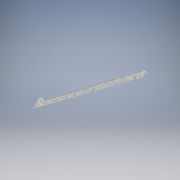
# Autodesk Inventor part: アーム先端1
Saved by Autodesk Inventor 2020 (Build 240168000, 168)
## iProperties
Created: 2018-11-26
Part Number: アーム先端1
Material: アルミニウム 7075
Document SubType Name: Modeling
Designer: 雪村
Density: 2.81 g/cm^3
Appearance: サテン - ブラシ仕上げ 重厚
Mass: 28.3471 g
Surface Area: 102.55 cm^2
Volume: 10.0879 cm^3
Description: アルミ7000 6t
Author: 雪村
Autodesk Inventor part; units mm, degrees
ref_plane "YZ Plane" through (0, 0, 0) normal (1, 0, 0) x (0, 1, 0)
ref_plane "XZ Plane" through (0, 0, 0) normal (0, 1, 0) x (-1, 0, 0)
ref_plane "XY Plane" through (0, 0, 0) normal (0, 0, 1) x (1, 0, 0)
sketch "スケッチ1" plane through (0, 0, 0) normal (0, 0, 1) x (1, 0, 0)
  line L0 (-218.2218, -75.2242) -> (-181.0358, -47.3081)
  line L1 (-181.0358, -47.3081) -> (-413.1791, -221.5813)
  line L2 (-39.9318, 79.9092) -> (-423.8001, -208.2662) construction
  arc A0 (-413.8727, -220.8729) -> (-413.1791, -221.5813) centre (-413.4792, -221.1815) ccw
  line L3 (-413.8727, -220.8729) -> (-401.6494, -205.2862)
  line L4 (-401.6494, -205.2862) -> (-186.2425, -41.2134)
  line L5 (-181.4863, -40.7689) -> (-171.6699, -53.845) construction
  line L6 (-423.8001, -208.2662) -> (-390.8364, -252.1761) construction
  circle A1 centre (-209.3341, -63.7077) radius 1.5
  circle A2 centre (-183.8101, -44.4068) radius 1.5
  arc A3 (-181.0358, -47.3081) -> (-186.2425, -41.2134) centre (-183.8101, -44.4068) ccw
  point P0 (0, 0)
  point P1 (0, 0)
  dimension "d0" = 1
  dimension "d1" = 15
  dimension "d2" = 8
  dimension "d3" = 0.4
  constraints: 14 end point, 4 centre point, 4 point on circle, 4 tangent, 1 parallel, 1 perpendicular, 6 other
  measures "d0" diameter of A0
  measures "d1" angle of L1 L3
  measures "d2" distance from line of L0 L4.end
  measures "d3" angle of L1 L4
extrude "押し出し1" add sketch "スケッチ1" along normal blind 6
sketch "スケッチ2" plane through (0, 0, 6) normal (0, 0, 1) x (1, 0, 0)
  circle A0 centre (-183.8101, -44.4068) radius 1.5 projected
  circle A1 centre (-209.3341, -63.7077) radius 1.5 projected
  line L0 (-413.1791, -221.5813) -> (-181.0358, -47.3081) projected
  arc A2 (-181.0358, -47.3081) -> (-186.2425, -41.2134) centre (-183.8101, -44.4068) ccw projected
  line L1 (-186.2425, -41.2134) -> (-401.6494, -205.2862) projected
  line L2 (-401.6494, -205.2862) -> (-413.8727, -220.8729) projected
  arc A3 (-413.8727, -220.8729) -> (-413.1791, -221.5813) centre (-413.4792, -221.1815) ccw projected
  line L3 (-183.8101, -44.4068) -> (-185.0065, -45.3115)
  line L4 (-209.7841, -65.1386) -> (-419.2967, -222.4226) construction
  line L5 (-413.1791, -221.5813) -> (-181.0358, -47.3081) projected
  circle A4 centre (-399.7939, -207.7816) radius 1.5
  circle A5 centre (-379.8007, -192.7724) radius 1.5
  circle A6 centre (-359.8076, -177.7633) radius 1.5
  circle A7 centre (-339.8144, -162.7542) radius 1.5
  circle A8 centre (-319.8213, -147.745) radius 1.5
  circle A9 centre (-299.8281, -132.7359) radius 1.5
  circle A10 centre (-399.7939, -207.7816) radius 3 construction
  line L6 (-401.6494, -205.2862) -> (-413.8727, -220.8729) projected
  circle A11 centre (-283.8336, -120.7286) radius 1.5
  circle A12 centre (-263.8405, -105.7194) radius 1.5
  circle A13 centre (-223.8542, -75.7012) radius 1.5
  circle A14 centre (-243.8473, -90.7103) radius 1.5
  point P0 (0, 0)
  dimension "d6" = 3
  dimension "d7" = 3
  dimension "d8" = 3
  dimension "d9" = 3
  dimension "d10" = 3
  dimension "d11" = 3
  dimension "d12" = 3
  dimension "d15" = 25
  dimension "d16" = 25
  dimension "d17" = 25
  dimension "d18" = 25
  dimension "d19" = 25
  dimension "d50" = 3
  dimension "d51" = 3
  dimension "d52" = 3
  dimension "d53" = 3
  dimension "d55" = 25
  dimension "d56" = 25
  dimension "d57" = 25
  dimension "d61" = 20
  constraints: 11 centre point, 2 end point, 2 tangent, 18 other
  measures "d7" diameter of A4
  measures "d8" diameter of A5
  measures "d9" diameter of A6
  measures "d10" diameter of A7
  measures "d11" diameter of A8
  measures "d12" diameter of A9
  measures "d15" distance of A5.centre A4.centre
  measures "d16" distance of A6.centre A5.centre
  measures "d17" distance of A7.centre A6.centre
  measures "d18" distance of A8.centre A7.centre
  measures "d19" distance of A8.centre A9.centre
  measures "d50" diameter of A11
  measures "d51" diameter of A12
  measures "d52" diameter of A13
  measures "d53" diameter of A14
  measures "d55" distance of A12.centre A11.centre
  measures "d56" distance of A14.centre A12.centre
  measures "d57" distance of A14.centre A13.centre
  measures "d61" distance of A9.centre A11.centre
extrude "押し出し2" cut sketch "スケッチ2" against normal blind 10 contours A4 | A5 | A6 | A7 | A8 | A9 | A11 | A12 | A13 | A14
sketch "スケッチ7" plane through (0, 0, 6) normal (0, 0, 1) x (1, 0, 0)
  line L0 (-413.1791, -221.5813) -> (-181.0358, -47.3081) construction
  arc A0 (-181.0358, -47.3081) -> (-186.2425, -41.2134) centre (-183.8101, -44.4068) ccw construction
  line L1 (-186.2425, -41.2134) -> (-401.6494, -205.2862) construction
  line L2 (-401.6494, -205.2862) -> (-413.8727, -220.8729) projected
  arc A1 (-413.8727, -220.8729) -> (-413.1791, -221.5813) centre (-413.4792, -221.1815) ccw projected
  circle A2 centre (-209.3341, -63.7077) radius 1.5 construction
  circle A3 centre (-183.8101, -44.4068) radius 1.5 construction
  line L3 (-186.2425, -41.2134) -> (-401.6494, -205.2862) projected
  line L4 (-401.6494, -205.2862) -> (-413.8727, -220.8729) projected
  line L5 (-413.9292, -220.9634) -> (-400.843, -193.968)
  arc A4 (-400.843, -193.968) -> (-394.0669, -199.5107) centre (-396.7936, -195.9309) ccw
  arc A5 (-413.8727, -220.8729) -> (-413.1791, -221.5813) centre (-413.4792, -221.1815) ccw projected
  point P0 (0, 0)
  dimension "d45" = 9
  dimension "d46" = 30
  constraints: 3 point on circle, 3 tangent, 2 end point, 1 centre point, 1 point on line
  measures "d45" diameter of A4
  measures "d46" distance of L5.start L5.end
extrude "押し出し6" add sketch "スケッチ7" against normal blind 6
fillet "フィレット3" radius 1 1 edges at (-400.843, -193.968, 3)
sketch "スケッチ13" plane through (0, 0, 6) normal (0, 0, 1) x (1, 0, 0)
  circle A0 centre (-183.8101, -44.4068) radius 1.5 construction
  circle A1 centre (-399.7939, -207.7816) radius 1.5 projected
  circle A2 centre (-183.8101, -44.4068) radius 1.5 construction
  line L0 (-185.6423, -44.4646) -> (-186.6877, -45.2549) construction
  circle A3 centre (-399.7939, -207.7816) radius 1.5 projected
  line L1 (-397.9939, -207.6808) -> (-396.933, -206.8784) construction
  line L2 (-185.6423, -44.4646) -> (-184.3878, -46.1357) construction
  line L3 (-413.1791, -221.5813) -> (-181.0358, -47.3081) construction
  line L4 (-399.2667, -205.9854) -> (-397.9939, -207.6808) construction
  line L5 (-186.2425, -41.2134) -> (-394.0669, -199.5107) construction
  line L6 (-394.0669, -199.5107) -> (-402.0801, -205.6142) construction
  circle A4 centre (-379.8007, -192.7724) radius 1.5 construction
  circle A5 centre (-359.8076, -177.7633) radius 1.5 construction
  circle A6 centre (-339.8144, -162.7542) radius 1.5 projected
  circle A7 centre (-319.8213, -147.745) radius 1.5 construction
  circle A8 centre (-299.8281, -132.7359) radius 1.5 projected
  circle A9 centre (-283.8336, -120.7286) radius 1.5 projected
  circle A10 centre (-263.8405, -105.7194) radius 1.5 construction
  circle A11 centre (-243.8473, -90.7103) radius 1.5 construction
  circle A12 centre (-223.8542, -75.7012) radius 1.5 construction
  circle A13 centre (-209.3341, -63.7077) radius 1.5 construction
  arc A14 (-397.9928, -210.1808) -> (-396.933, -206.8784) centre (-399.7939, -207.7816) ccw construction
  arc A15 (-376.9695, -191.7805) -> (-378.3319, -190.1566) centre (-379.8007, -192.7724) ccw
  arc A16 (-362.7452, -178.3716) -> (-361.608, -180.163) centre (-359.8076, -177.7633) ccw
  arc A17 (-342.77, -163.2684) -> (-341.6875, -165.0976) centre (-339.8144, -162.7542) ccw
  arc A18 (-317.093, -146.4974) -> (-318.6095, -145.0007) centre (-319.8213, -147.745) ccw
  arc A19 (-298.027, -135.1351) -> (-297.1388, -131.4065) centre (-299.8281, -132.7359) ccw construction
  arc A20 (-286.8241, -120.9678) -> (-285.898, -122.9054) centre (-283.8336, -120.7286) ccw
  arc A21 (-266.8374, -105.8559) -> (-265.969, -107.8336) centre (-263.8405, -105.7194) ccw
  arc A22 (-246.8472, -90.7414) -> (-246.0378, -92.7601) centre (-243.8473, -90.7103) ccw
  arc A23 (-226.8532, -75.624) -> (-226.1046, -77.6851) centre (-223.8542, -75.7012) ccw
  arc A24 (-212.2122, -64.554) -> (-210.958, -66.2301) centre (-209.3341, -63.7077) ccw
  arc A25 (-186.6877, -45.2549) -> (-185.4357, -46.9282) centre (-183.8101, -44.4068) ccw
  line L7 (-398.2446, -205.2126) -> (-399.2667, -205.9854) construction
  arc A26 (-398.2446, -205.2126) -> (-397.9928, -210.1808) centre (-399.7939, -207.7816) ccw construction
  line L8 (-396.933, -206.8784) -> (-381.5261, -195.2266)
  arc A27 (-396.933, -206.8784) -> (-398.2446, -205.2126) centre (-399.7939, -207.7816) ccw
  line L9 (-382.7178, -193.4728) -> (-398.2446, -205.2126)
  line L10 (-381.5261, -195.2266) -> (-376.9695, -191.7805) construction
  arc A28 (-377.9996, -195.1716) -> (-376.9695, -191.7805) centre (-379.8007, -192.7724) ccw construction
  line L11 (-378.3319, -190.1566) -> (-382.7178, -193.4728) construction
  arc A29 (-382.7178, -193.4728) -> (-381.5261, -195.2266) centre (-379.8007, -192.7724) ccw
  arc A30 (-378.3319, -190.1566) -> (-382.7178, -193.4728) centre (-379.8007, -192.7724) ccw construction
  line L12 (-376.9695, -191.7805) -> (-361.608, -180.163)
  arc A31 (-381.5261, -195.2266) -> (-377.9996, -195.1716) centre (-379.8007, -192.7724) ccw construction
  arc A32 (-358.4217, -175.1026) -> (-362.7452, -178.3716) centre (-359.8076, -177.7633) ccw construction
  arc A33 (-361.608, -180.163) -> (-357.0083, -176.6844) centre (-359.8076, -177.7633) ccw construction
  line L13 (-357.0083, -176.6844) -> (-341.6875, -165.0976)
  arc A34 (-357.0083, -176.6844) -> (-358.4217, -175.1026) centre (-359.8076, -177.7633) ccw
  line L14 (-358.4217, -175.1026) -> (-362.7452, -178.3716) construction
  line L15 (-362.7452, -178.3716) -> (-378.3319, -190.1566)
  line L16 (-361.608, -180.163) -> (-358.3105, -177.6692) construction
  line L17 (-358.3105, -177.6692) -> (-357.0083, -176.6844) construction
  arc A35 (-338.5142, -160.0506) -> (-342.77, -163.2684) centre (-339.8144, -162.7542) ccw construction
  line L18 (-337.0495, -161.59) -> (-321.7647, -150.0305)
  line L19 (-341.6875, -165.0976) -> (-337.0495, -161.59) construction
  arc A36 (-337.0495, -161.59) -> (-338.5142, -160.0506) centre (-339.8144, -162.7542) ccw
  arc A37 (-341.6875, -165.0976) -> (-337.0495, -161.59) centre (-339.8144, -162.7542) ccw construction
  line L20 (-338.5142, -160.0506) -> (-342.77, -163.2684) construction
  line L21 (-342.77, -163.2684) -> (-358.4217, -175.1026)
  line L22 (-322.792, -148.1631) -> (-338.5142, -160.0506)
  line L23 (-318.6095, -145.0007) -> (-322.792, -148.1631) construction
  arc A38 (-318.0202, -150.1442) -> (-317.093, -146.4974) centre (-319.8213, -147.745) ccw construction
  line L24 (-321.7647, -150.0305) -> (-317.093, -146.4974) construction
  line L25 (-317.093, -146.4974) -> (-301.8396, -134.9616)
  arc A39 (-321.7647, -150.0305) -> (-318.0202, -150.1442) centre (-319.8213, -147.745) ccw construction
  arc A40 (-318.6095, -145.0007) -> (-322.792, -148.1631) centre (-319.8213, -147.745) ccw construction
  arc A41 (-322.792, -148.1631) -> (-321.7647, -150.0305) centre (-319.8213, -147.745) ccw
  line L26 (-302.8111, -133.0555) -> (-318.6095, -145.0007)
  line L27 (-298.7077, -129.953) -> (-302.8111, -133.0555) construction
  line L28 (-297.1388, -131.4065) -> (-285.898, -122.9054)
  line L29 (-301.8396, -134.9616) -> (-297.1388, -131.4065) construction
  arc A42 (-301.8396, -134.9616) -> (-298.027, -135.1351) centre (-299.8281, -132.7359) ccw construction
  arc A43 (-297.1388, -131.4065) -> (-298.7077, -129.953) centre (-299.8281, -132.7359) ccw
  arc A44 (-298.7077, -129.953) -> (-302.8111, -133.0555) centre (-299.8281, -132.7359) ccw construction
  arc A45 (-302.8111, -133.0555) -> (-301.8396, -134.9616) centre (-299.8281, -132.7359) ccw
  arc A46 (-282.7885, -117.9165) -> (-286.8241, -120.9678) centre (-283.8336, -120.7286) ccw construction
  line L30 (-286.8241, -120.9678) -> (-298.7077, -129.953)
  line L31 (-282.7885, -117.9165) -> (-286.8241, -120.9678) construction
  line L32 (-281.177, -119.335) -> (-265.969, -107.8336)
  line L33 (-285.898, -122.9054) -> (-281.177, -119.335) construction
  arc A47 (-285.898, -122.9054) -> (-281.177, -119.335) centre (-283.8336, -120.7286) ccw construction
  arc A48 (-281.177, -119.335) -> (-282.7885, -117.9165) centre (-283.8336, -120.7286) ccw
  arc A49 (-262.8925, -102.8732) -> (-266.8374, -105.8559) centre (-263.8405, -105.7194) ccw construction
  arc A50 (-261.2267, -104.2471) -> (-262.8925, -102.8732) centre (-263.8405, -105.7194) ccw
  arc A51 (-265.969, -107.8336) -> (-261.2267, -104.2471) centre (-263.8405, -105.7194) ccw construction
  line L34 (-265.969, -107.8336) -> (-261.2267, -104.2471) construction
  line L35 (-261.2267, -104.2471) -> (-246.0378, -92.7601)
  line L36 (-262.8925, -102.8732) -> (-266.8374, -105.8559) construction
  line L37 (-266.8374, -105.8559) -> (-282.7885, -117.9165)
  arc A52 (-242.9999, -87.8325) -> (-246.8472, -90.7414) centre (-243.8473, -90.7103) ccw construction
  arc A53 (-246.0378, -92.7601) -> (-241.2785, -89.1608) centre (-243.8473, -90.7103) ccw construction
  arc A54 (-241.2785, -89.1608) -> (-242.9999, -87.8325) centre (-243.8473, -90.7103) ccw
  line L38 (-241.2785, -89.1608) -> (-226.1046, -77.6851)
  line L39 (-246.0378, -92.7601) -> (-241.2785, -89.1608) construction
  line L40 (-246.8472, -90.7414) -> (-262.8925, -102.8732)
  line L41 (-242.9999, -87.8325) -> (-246.8472, -90.7414) construction
  arc A55 (-223.1112, -72.7946) -> (-226.8532, -75.624) centre (-223.8542, -75.7012) ccw construction
  arc A56 (-226.1046, -77.6851) -> (-221.3325, -74.0761) centre (-223.8542, -75.7012) ccw construction
  arc A57 (-221.3325, -74.0761) -> (-223.1112, -72.7946) centre (-223.8542, -75.7012) ccw
  line L42 (-221.3325, -74.0761) -> (-210.958, -66.2301)
  line L43 (-223.1112, -72.7946) -> (-226.8532, -75.624) construction
  line L44 (-226.8532, -75.624) -> (-242.9999, -87.8325)
  line L45 (-224.9014, -76.7751) -> (-221.3325, -74.0761) construction
  line L46 (-226.1046, -77.6851) -> (-224.9014, -76.7751) construction
  arc A58 (-207.7355, -61.1691) -> (-212.2122, -64.554) centre (-209.3341, -63.7077) ccw construction
  arc A59 (-210.958, -66.2301) -> (-206.4647, -62.832) centre (-209.3341, -63.7077) ccw construction
  arc A60 (-206.4647, -62.832) -> (-207.7355, -61.1691) centre (-209.3341, -63.7077) ccw
  line L47 (-206.4647, -62.832) -> (-185.4357, -46.9282)
  line L48 (-210.958, -66.2301) -> (-206.4647, -62.832) construction
  line L49 (-212.2122, -64.554) -> (-223.1112, -72.7946)
  line L50 (-207.7355, -61.1691) -> (-212.2122, -64.554) construction
  arc A61 (-185.4357, -46.9282) -> (-183.4499, -47.3851) centre (-183.8101, -44.4068) ccw construction
  line L51 (-186.6877, -45.2549) -> (-207.7355, -61.1691)
  line L52 (-185.4357, -46.9282) -> (-184.3878, -46.1357) construction
  arc A62 (-183.4499, -47.3851) -> (-186.6877, -45.2549) centre (-183.8101, -44.4068) ccw construction
  point P0 (0, 0)
  dimension "d70" = 2
  dimension "d71" = 2.95
  dimension "d72" = 2.95
  dimension "d73" = 2
  dimension "d74" = 1.5
  dimension "d75" = 1.5
  dimension "d76" = 1.5
  dimension "d77" = 1.5
  dimension "d78" = 1.5
  dimension "d79" = 1.5
  dimension "d80" = 1.5
  dimension "d81" = 1.5
  dimension "d82" = 1.5
  dimension "d83" = 1.5
  dimension "d84" = 1.5
  dimension "d85" = 1.5
  constraints: 108 point on circle, 102 end point, 49 centre point, 47 collinear, 11 point on line, 2 perpendicular, 2 tangent, 4 other
  measures "d70" distance from line of L3 L1.start
  measures "d71" distance from line of L3 L2.end
  measures "d72" distance from line of L0.start L5
  measures "d73" distance from line of L6 L4.start
  measures "d74" radial gap between concentric circles of A1 A14
  measures "d75" radial gap between concentric circles of A4 A15
  measures "d77" radial gap between concentric circles of A6 A17
  measures "d78" radial gap between concentric circles of A7 A18
  measures "d79" radial gap between concentric circles of A8 A19
  measures "d80" radial gap between concentric circles of A9 A20
  measures "d81" radial gap between concentric circles of A10 A21
  measures "d82" radial gap between concentric circles of A11 A22
  measures "d84" radial gap between concentric circles of A13 A24
  measures "d85" radial gap between concentric circles of A2 A25
extrude "押し出し11" cut sketch "スケッチ13" against normal through all contours A15 L15 A16 L12 | A17 L13 A34 L21 | A18 L26 A45 L25 | A20 L28 A43 L30 | A21 L32 A48 L37 | A22 L35 A50 L40 | A23 L38 A54 L44 | A24 L42 A57 L49 | A25 L47 A60 L51 | A27 L9 A29 L8 | A36 L22 A41 L18
fillet "フィレット4" radius 1 44 edges at (-398.2446, -205.2126, 3) (-382.7178, -193.4728, 3) (-396.933, -206.8784, 3) (-381.5261, -195.2266, 3) (-376.9695, -191.7805, 3) (-361.608, -180.163, 3) (-362.7452, -178.3716, 3) (-378.3319, -190.1566, 3) (-358.4217, -175.1026, 3) (-342.77, -163.2684, 3) (-357.0083, -176.6844, 3) (-341.6875, -165.0976, 3) (-338.5142, -160.0506, 3) (-322.792, -148.1631, 3) (-337.0495, -161.59, 3) (-321.7647, -150.0305, 3) (-318.6095, -145.0007, 3) (-302.8111, -133.0555, 3) (-317.093, -146.4974, 3) (-301.8396, -134.9616, 3) (-298.7077, -129.953, 3) (-286.8241, -120.9678, 3) (-297.1388, -131.4065, 3) (-285.898, -122.9054, 3) (-282.7885, -117.9165, 3) (-266.8374, -105.8559, 3) (-281.177, -119.335, 3) (-265.969, -107.8336, 3) (-262.8925, -102.8732, 3) (-246.8472, -90.7414, 3) (-261.2267, -104.2471, 3) (-246.0378, -92.7601, 3) (-242.9999, -87.8325, 3) (-226.8532, -75.624, 3) (-241.2785, -89.1608, 3) (-226.1046, -77.6851, 3) (-223.1112, -72.7946, 3) (-212.2122, -64.554, 3) (-221.3325, -74.0761, 3) (-210.958, -66.2301, 3) (-207.7355, -61.1691, 3) (-186.6877, -45.2549, 3) (-206.4647, -62.832, 3) (-185.4357, -46.9282, 3)
sketch "スケッチ14" plane through (0, 0, 0) normal (0, 0, -1) x (-1, 0, 0)
  line L0 (376.0581, -191.0913) -> (362.4956, -180.8342) projected
  arc A0 (362.276, -179.4683) -> (362.4956, -180.8342) centre (363.0988, -180.0366) ccw projected
  arc A1 (362.276, -179.4683) -> (362.324, -179.3966) centre (359.8076, -177.7633) ccw projected
  arc A2 (363.7659, -179.1433) -> (362.324, -179.3966) centre (363.1628, -179.941) ccw projected
  line L1 (363.7659, -179.1433) -> (377.3382, -189.4053) projected
  arc A3 (377.5015, -190.8454) -> (377.3382, -189.4053) centre (376.7351, -190.203) ccw projected
  arc A4 (377.5015, -190.8454) -> (377.4462, -190.9134) centre (379.8007, -192.7724) ccw projected
  arc A5 (376.0581, -191.0913) -> (377.4462, -190.9134) centre (376.6613, -190.2937) ccw projected
  line L2 (205.5211, -62.1183) -> (186.3788, -47.6414) projected
  arc A6 (186.189, -46.2346) -> (186.3788, -47.6414) centre (186.9819, -46.8438) ccw projected
  line L3 (187.639, -45.9743) -> (206.7836, -60.4494) projected
  arc A7 (206.9689, -61.8622) -> (206.7836, -60.4494) centre (206.1805, -61.2471) ccw projected
  arc A8 (206.9689, -61.8622) -> (206.9268, -61.9175) centre (209.3341, -63.7077) ccw projected
  arc A9 (205.5211, -62.1183) -> (206.9268, -61.9175) centre (206.1243, -61.3208) ccw projected
  line L4 (316.2507, -145.8604) -> (302.6604, -135.5823) projected
  arc A10 (302.4047, -134.2725) -> (302.6604, -135.5823) centre (303.2636, -134.7848) ccw projected
  arc A11 (302.4047, -134.2725) -> (302.445, -134.2029) centre (299.8281, -132.7359) ccw projected
  arc A12 (303.9204, -133.8943) -> (302.445, -134.2029) centre (303.3172, -134.6919) ccw projected
  line L5 (303.9204, -133.8943) -> (317.5311, -144.1853) projected
  arc A13 (317.6513, -145.6735) -> (317.5311, -144.1853) centre (316.928, -144.983) ccw projected
  arc A14 (317.6513, -145.6735) -> (317.5957, -145.7333) centre (319.8213, -147.745) ccw projected
  arc A15 (316.2507, -145.8604) -> (317.5957, -145.7333) centre (316.8539, -145.0628) ccw projected
  line L6 (260.4433, -103.6546) -> (246.8012, -93.3374) projected
  arc A16 (246.5151, -92.0825) -> (246.8012, -93.3374) centre (247.4044, -92.5399) ccw projected
  arc A17 (246.5151, -92.0825) -> (246.5487, -92.0152) centre (243.8473, -90.7103) ccw projected
  arc A18 (248.0522, -91.6525) -> (246.5487, -92.0152) centre (247.4491, -92.4502) ccw projected
  line L7 (248.0522, -91.6525) -> (261.7233, -101.9892) projected
  arc A19 (261.8003, -103.52) -> (261.7233, -101.9892) centre (261.1202, -102.7869) ccw projected
  arc A20 (261.8003, -103.52) -> (261.745, -103.5726) centre (263.8405, -105.7194) ccw projected
  arc A21 (260.4433, -103.6546) -> (261.745, -103.5726) centre (261.0465, -102.857) ccw projected
  line L8 (296.318, -130.7858) -> (286.7019, -123.5134) projected
  arc A22 (286.4372, -122.219) -> (286.7019, -123.5134) centre (287.3051, -122.7158) ccw projected
  arc A23 (286.4372, -122.219) -> (286.4755, -122.15) centre (283.8336, -120.7286) ccw projected
  arc A24 (287.9593, -121.8261) -> (286.4755, -122.15) centre (287.3561, -122.6238) ccw projected
  line L9 (287.9593, -121.8261) -> (297.5984, -129.1142) projected
  arc A25 (297.7035, -130.6179) -> (297.5984, -129.1142) centre (296.9953, -129.9119) ccw projected
  arc A26 (297.7035, -130.6179) -> (297.6479, -130.6751) centre (299.8281, -132.7359) ccw projected
  arc A27 (296.318, -130.7858) -> (297.6479, -130.6751) centre (296.9212, -129.9882) ccw projected
  line L10 (220.5886, -73.5135) -> (211.9017, -66.9438) projected
  arc A28 (211.7122, -65.5366) -> (211.9017, -66.9438) centre (212.5049, -66.1462) ccw projected
  arc A29 (211.7122, -65.5366) -> (211.7543, -65.4804) centre (209.3341, -63.7077) ccw projected
  arc A30 (213.1641, -65.2737) -> (211.7543, -65.4804) centre (212.561, -66.0714) ccw projected
  line L11 (213.1641, -65.2737) -> (221.868, -71.8547) projected
  arc A31 (221.9122, -73.4145) -> (221.868, -71.8547) centre (221.2649, -72.6523) ccw projected
  arc A32 (221.9122, -73.4145) -> (221.8574, -73.4622) centre (223.8542, -75.7012) ccw projected
  arc A33 (220.5886, -73.5135) -> (221.8574, -73.4622) centre (221.1918, -72.7159) ccw projected
  line L12 (240.5151, -88.5834) -> (226.8484, -78.2476) projected
  arc A34 (226.5523, -77.0128) -> (226.8484, -78.2476) centre (227.4516, -77.45) ccw projected
  arc A35 (226.5523, -77.0128) -> (226.5835, -76.9465) centre (223.8542, -75.7012) ccw projected
  arc A36 (228.0964, -76.564) -> (226.5835, -76.9465) centre (227.4933, -77.3616) ccw projected
  line L13 (228.0964, -76.564) -> (241.7949, -86.9213) projected
  arc A37 (241.8556, -88.4668) -> (241.7949, -86.9213) centre (241.1918, -87.719) ccw projected
  arc A38 (241.8556, -88.4668) -> (241.8006, -88.517) centre (243.8473, -90.7103) ccw projected
  arc A39 (240.5151, -88.5834) -> (241.8006, -88.517) centre (241.1183, -87.7858) ccw projected
  line L14 (280.373, -118.727) -> (266.7524, -108.426) projected
  arc A40 (266.4768, -107.1512) -> (266.7524, -108.426) centre (267.3556, -107.6284) ccw projected
  arc A41 (266.4768, -107.1512) -> (266.5127, -107.083) centre (263.8405, -105.7194) ccw projected
  arc A42 (268.0065, -106.7399) -> (266.5127, -107.083) centre (267.4034, -107.5376) ccw projected
  line L15 (268.0065, -106.7399) -> (281.6533, -117.0582) projected
  arc A43 (281.746, -118.574) -> (281.6533, -117.0582) centre (281.0502, -117.8559) ccw projected
  arc A44 (281.746, -118.574) -> (281.6906, -118.6292) centre (283.8336, -120.7286) ccw projected
  arc A45 (280.373, -118.727) -> (281.6906, -118.6292) centre (280.9762, -117.9294) ccw projected
  line L16 (336.1849, -160.9361) -> (322.607, -150.6675) projected
  arc A46 (322.363, -149.3387) -> (322.607, -150.6675) centre (323.2102, -149.8699) ccw projected
  arc A47 (322.363, -149.3387) -> (322.4058, -149.2683) centre (319.8213, -147.745) ccw projected
  arc A48 (323.8704, -148.9784) -> (322.4058, -149.2683) centre (323.2673, -149.7761) ccw projected
  line L17 (323.8704, -148.9784) -> (337.4653, -159.2575) projected
  arc A49 (337.6003, -160.7299) -> (337.4653, -159.2575) centre (336.8622, -160.0552) ccw projected
  arc A50 (337.6003, -160.7299) -> (337.5447, -160.7925) centre (339.8144, -162.7542) ccw projected
  arc A51 (336.1849, -160.9361) -> (337.5447, -160.7925) centre (336.7881, -160.1386) ccw projected
  line L18 (356.1207, -176.0131) -> (342.5521, -165.7515) projected
  arc A52 (342.3201, -164.4039) -> (342.5521, -165.7515) centre (343.1553, -164.9539) ccw projected
  arc A53 (342.3201, -164.4039) -> (342.3654, -164.3329) centre (339.8144, -162.7542) ccw projected
  arc A54 (343.8189, -164.0615) -> (342.3654, -164.3329) centre (343.2158, -164.8591) ccw projected
  line L19 (343.8189, -164.0615) -> (357.401, -174.3309) projected
  arc A55 (357.5503, -175.7872) -> (357.401, -174.3309) centre (356.7979, -175.1285) ccw projected
  arc A56 (357.5503, -175.7872) -> (357.4948, -175.8525) centre (359.8076, -177.7633) ccw projected
  arc A57 (356.1207, -176.0131) -> (357.4948, -175.8525) centre (356.7239, -175.2155) ccw projected
  line L20 (395.9971, -206.1706) -> (382.4375, -195.9158) projected
  arc A58 (382.2307, -194.5318) -> (382.4375, -195.9158) centre (383.0407, -195.1182) ccw projected
  arc A59 (382.2307, -194.5318) -> (382.2814, -194.4594) centre (379.8007, -192.7724) ccw projected
  arc A60 (383.7115, -194.2241) -> (382.2814, -194.4594) centre (383.1083, -195.0218) ccw projected
  line L21 (383.7115, -194.2241) -> (397.2769, -204.4809) projected
  arc A61 (397.4538, -205.9043) -> (397.2769, -204.4809) centre (396.6738, -205.2786) ccw projected
  arc A62 (397.4538, -205.9043) -> (397.3987, -205.9752) centre (399.7939, -207.7816) ccw projected
  arc A63 (395.9971, -206.1706) -> (397.3987, -205.9752) centre (396.6003, -205.373) ccw projected
  arc A64 (402.6936, -197.7857) -> (400.8847, -197.8054) centre (401.7938, -198.2219) ccw projected
  arc A65 (394.0669, -199.5107) -> (400.8847, -197.8054) centre (396.7936, -195.9309) ccw projected
  line L22 (394.0669, -199.5107) -> (186.2425, -41.2134) projected
  arc A66 (186.2425, -41.2134) -> (181.0358, -47.3081) centre (183.8101, -44.4068) ccw projected
  line L23 (181.0358, -47.3081) -> (413.1791, -221.5813) projected
  arc A67 (413.1791, -221.5813) -> (413.9292, -220.9634) centre (413.4792, -221.1815) ccw projected
  line L24 (413.9292, -220.9634) -> (402.6936, -197.7857) projected
  circle A68 centre (223.8542, -75.7012) radius 1.5 projected
  circle A69 centre (283.8336, -120.7286) radius 1.5 projected
  circle A70 centre (319.8213, -147.745) radius 1.5 projected
  circle A71 centre (359.8076, -177.7633) radius 1.5 projected
  circle A72 centre (399.7939, -207.7816) radius 1.5 projected
  circle A73 centre (379.8007, -192.7724) radius 1.5 projected
  circle A74 centre (339.8144, -162.7542) radius 1.5 projected
  circle A75 centre (299.8281, -132.7359) radius 1.5 projected
  circle A76 centre (263.8405, -105.7194) radius 1.5 projected
  circle A77 centre (243.8473, -90.7103) radius 1.5 projected
  circle A78 centre (183.8101, -44.4068) radius 1.5 projected
  circle A79 centre (209.3341, -63.7077) radius 1.5 projected
  arc A80 (186.189, -46.2346) -> (186.2295, -46.1806) centre (183.8101, -44.4068) ccw projected
  arc A81 (187.639, -45.9743) -> (186.2295, -46.1806) centre (187.0359, -46.7719) ccw projected
  point P0 (0, 0)
extrude "押し出し12" add sketch "スケッチ14" against normal blind 1.5 contours L0 A0 A1 A2 L1 A3 A4 A5 | L2 A6 A80 A81 L3 A7 A8 A9 | L4 A10 A11 A12 L5 A13 A14 A15 | L6 A16 A17 A18 L7 A19 A20 A21 | L8 A22 A23 A24 L9 A25 A26 A27 | L10 A28 A29 A30 L11 A31 A32 A33 | L12 A34 A35 A36 L13 A37 A38 A39 | L14 A40 A41 A42 L15 A43 A44 A45 | L16 A46 A47 A48 L17 A49 A50 A51 | L18 A52 A53 A54 L19 A55 A56 A57 | L20 A58 A59 A60 L21 A61 A62 A63
sketch "スケッチ15" plane through (0, 0, 6) normal (0, 0, 1) x (1, 0, 0)
  line L0 (-362.4956, -180.8342) -> (-376.0581, -191.0913) projected
  arc A0 (-377.4462, -190.9134) -> (-376.0581, -191.0913) centre (-376.6613, -190.2937) ccw projected
  arc A1 (-377.4462, -190.9134) -> (-377.5015, -190.8454) centre (-379.8007, -192.7724) ccw projected
  arc A2 (-377.3382, -189.4053) -> (-377.5015, -190.8454) centre (-376.7351, -190.203) ccw projected
  line L1 (-377.3382, -189.4053) -> (-363.7659, -179.1433) projected
  arc A3 (-362.324, -179.3966) -> (-363.7659, -179.1433) centre (-363.1628, -179.941) ccw projected
  arc A4 (-362.324, -179.3966) -> (-362.276, -179.4683) centre (-359.8076, -177.7633) ccw projected
  arc A5 (-362.4956, -180.8342) -> (-362.276, -179.4683) centre (-363.0988, -180.0366) ccw projected
  line L2 (-186.3788, -47.6414) -> (-205.5211, -62.1183) projected
  arc A6 (-206.9268, -61.9175) -> (-205.5211, -62.1183) centre (-206.1243, -61.3208) ccw projected
  arc A7 (-206.9268, -61.9175) -> (-206.9689, -61.8622) centre (-209.3341, -63.7077) ccw projected
  arc A8 (-206.7836, -60.4494) -> (-206.9689, -61.8622) centre (-206.1805, -61.2471) ccw projected
  line L3 (-206.7836, -60.4494) -> (-187.639, -45.9743) projected
  arc A9 (-186.2295, -46.1806) -> (-187.639, -45.9743) centre (-187.0359, -46.7719) ccw projected
  arc A10 (-186.2295, -46.1806) -> (-186.189, -46.2346) centre (-183.8101, -44.4068) ccw projected
  arc A11 (-186.3788, -47.6414) -> (-186.189, -46.2346) centre (-186.9819, -46.8438) ccw projected
  line L4 (-302.6604, -135.5823) -> (-316.2507, -145.8604) projected
  arc A12 (-317.5957, -145.7333) -> (-316.2507, -145.8604) centre (-316.8539, -145.0628) ccw projected
  arc A13 (-317.5957, -145.7333) -> (-317.6513, -145.6735) centre (-319.8213, -147.745) ccw projected
  arc A14 (-317.5311, -144.1853) -> (-317.6513, -145.6735) centre (-316.928, -144.983) ccw projected
  line L5 (-317.5311, -144.1853) -> (-303.9204, -133.8943) projected
  arc A15 (-302.445, -134.2029) -> (-303.9204, -133.8943) centre (-303.3172, -134.6919) ccw projected
  arc A16 (-302.445, -134.2029) -> (-302.4047, -134.2725) centre (-299.8281, -132.7359) ccw projected
  arc A17 (-302.6604, -135.5823) -> (-302.4047, -134.2725) centre (-303.2636, -134.7848) ccw projected
  line L6 (-246.8012, -93.3374) -> (-260.4433, -103.6546) projected
  arc A18 (-261.745, -103.5726) -> (-260.4433, -103.6546) centre (-261.0465, -102.857) ccw projected
  arc A19 (-261.745, -103.5726) -> (-261.8003, -103.52) centre (-263.8405, -105.7194) ccw projected
  arc A20 (-261.7233, -101.9892) -> (-261.8003, -103.52) centre (-261.1202, -102.7869) ccw projected
  line L7 (-261.7233, -101.9892) -> (-248.0522, -91.6525) projected
  arc A21 (-246.5487, -92.0152) -> (-248.0522, -91.6525) centre (-247.4491, -92.4502) ccw projected
  arc A22 (-246.5487, -92.0152) -> (-246.5151, -92.0825) centre (-243.8473, -90.7103) ccw projected
  arc A23 (-246.8012, -93.3374) -> (-246.5151, -92.0825) centre (-247.4044, -92.5399) ccw projected
  line L8 (-286.7019, -123.5134) -> (-296.318, -130.7858) projected
  arc A24 (-297.6479, -130.6751) -> (-296.318, -130.7858) centre (-296.9212, -129.9882) ccw projected
  arc A25 (-297.6479, -130.6751) -> (-297.7035, -130.6179) centre (-299.8281, -132.7359) ccw projected
  arc A26 (-297.5984, -129.1142) -> (-297.7035, -130.6179) centre (-296.9953, -129.9119) ccw projected
  line L9 (-297.5984, -129.1142) -> (-287.9593, -121.8261) projected
  arc A27 (-286.4755, -122.15) -> (-287.9593, -121.8261) centre (-287.3561, -122.6238) ccw projected
  arc A28 (-286.4755, -122.15) -> (-286.4372, -122.219) centre (-283.8336, -120.7286) ccw projected
  arc A29 (-286.7019, -123.5134) -> (-286.4372, -122.219) centre (-287.3051, -122.7158) ccw projected
  line L10 (-211.9017, -66.9438) -> (-220.5886, -73.5135) projected
  arc A30 (-221.8574, -73.4622) -> (-220.5886, -73.5135) centre (-221.1918, -72.7159) ccw projected
  arc A31 (-221.8574, -73.4622) -> (-221.9122, -73.4145) centre (-223.8542, -75.7012) ccw projected
  arc A32 (-221.868, -71.8547) -> (-221.9122, -73.4145) centre (-221.2649, -72.6523) ccw projected
  line L11 (-221.868, -71.8547) -> (-213.1641, -65.2737) projected
  arc A33 (-211.7543, -65.4804) -> (-213.1641, -65.2737) centre (-212.561, -66.0714) ccw projected
  arc A34 (-211.7543, -65.4804) -> (-211.7122, -65.5366) centre (-209.3341, -63.7077) ccw projected
  arc A35 (-211.9017, -66.9438) -> (-211.7122, -65.5366) centre (-212.5049, -66.1462) ccw projected
  line L12 (-226.8484, -78.2476) -> (-240.5151, -88.5834) projected
  arc A36 (-241.8006, -88.517) -> (-240.5151, -88.5834) centre (-241.1183, -87.7858) ccw projected
  arc A37 (-241.8006, -88.517) -> (-241.8556, -88.4668) centre (-243.8473, -90.7103) ccw projected
  arc A38 (-241.7949, -86.9213) -> (-241.8556, -88.4668) centre (-241.1918, -87.719) ccw projected
  line L13 (-241.7949, -86.9213) -> (-228.0964, -76.564) projected
  arc A39 (-226.5835, -76.9465) -> (-228.0964, -76.564) centre (-227.4933, -77.3616) ccw projected
  arc A40 (-226.5835, -76.9465) -> (-226.5523, -77.0128) centre (-223.8542, -75.7012) ccw projected
  arc A41 (-226.8484, -78.2476) -> (-226.5523, -77.0128) centre (-227.4516, -77.45) ccw projected
  line L14 (-266.7524, -108.426) -> (-280.373, -118.727) projected
  arc A42 (-281.6906, -118.6292) -> (-280.373, -118.727) centre (-280.9762, -117.9294) ccw projected
  arc A43 (-281.6906, -118.6292) -> (-281.746, -118.574) centre (-283.8336, -120.7286) ccw projected
  arc A44 (-281.6533, -117.0582) -> (-281.746, -118.574) centre (-281.0502, -117.8559) ccw projected
  line L15 (-281.6533, -117.0582) -> (-268.0065, -106.7399) projected
  arc A45 (-266.5127, -107.083) -> (-268.0065, -106.7399) centre (-267.4034, -107.5376) ccw projected
  arc A46 (-266.5127, -107.083) -> (-266.4768, -107.1512) centre (-263.8405, -105.7194) ccw projected
  arc A47 (-266.7524, -108.426) -> (-266.4768, -107.1512) centre (-267.3556, -107.6284) ccw projected
  line L16 (-322.607, -150.6675) -> (-336.1849, -160.9361) projected
  arc A48 (-337.5447, -160.7925) -> (-336.1849, -160.9361) centre (-336.7881, -160.1386) ccw projected
  arc A49 (-337.5447, -160.7925) -> (-337.6003, -160.7299) centre (-339.8144, -162.7542) ccw projected
  arc A50 (-337.4653, -159.2575) -> (-337.6003, -160.7299) centre (-336.8622, -160.0552) ccw projected
  line L17 (-337.4653, -159.2575) -> (-323.8704, -148.9784) projected
  arc A51 (-322.4058, -149.2683) -> (-323.8704, -148.9784) centre (-323.2673, -149.7761) ccw projected
  arc A52 (-322.4058, -149.2683) -> (-322.363, -149.3387) centre (-319.8213, -147.745) ccw projected
  arc A53 (-322.607, -150.6675) -> (-322.363, -149.3387) centre (-323.2102, -149.8699) ccw projected
  line L18 (-342.5521, -165.7515) -> (-356.1207, -176.0131) projected
  arc A54 (-357.4948, -175.8525) -> (-356.1207, -176.0131) centre (-356.7239, -175.2155) ccw projected
  arc A55 (-357.4948, -175.8525) -> (-357.5503, -175.7872) centre (-359.8076, -177.7633) ccw projected
  arc A56 (-357.401, -174.3309) -> (-357.5503, -175.7872) centre (-356.7979, -175.1285) ccw projected
  line L19 (-357.401, -174.3309) -> (-343.8189, -164.0615) projected
  arc A57 (-342.3654, -164.3329) -> (-343.8189, -164.0615) centre (-343.2158, -164.8591) ccw projected
  arc A58 (-342.3654, -164.3329) -> (-342.3201, -164.4039) centre (-339.8144, -162.7542) ccw projected
  arc A59 (-342.5521, -165.7515) -> (-342.3201, -164.4039) centre (-343.1553, -164.9539) ccw projected
  line L20 (-382.4375, -195.9158) -> (-395.9971, -206.1706) projected
  arc A60 (-397.3987, -205.9752) -> (-395.9971, -206.1706) centre (-396.6003, -205.373) ccw projected
  arc A61 (-397.3987, -205.9752) -> (-397.4538, -205.9043) centre (-399.7939, -207.7816) ccw projected
  arc A62 (-397.2769, -204.4809) -> (-397.4538, -205.9043) centre (-396.6738, -205.2786) ccw projected
  line L21 (-397.2769, -204.4809) -> (-383.7115, -194.2241) projected
  arc A63 (-382.2814, -194.4594) -> (-383.7115, -194.2241) centre (-383.1083, -195.0218) ccw projected
  arc A64 (-382.2814, -194.4594) -> (-382.2307, -194.5318) centre (-379.8007, -192.7724) ccw projected
  arc A65 (-382.4375, -195.9158) -> (-382.2307, -194.5318) centre (-383.0407, -195.1182) ccw projected
  arc A66 (-400.8847, -197.8054) -> (-402.6936, -197.7857) centre (-401.7938, -198.2219) ccw projected
  line L22 (-413.9292, -220.9634) -> (-402.6936, -197.7857) projected
  arc A67 (-413.9292, -220.9634) -> (-413.1791, -221.5813) centre (-413.4792, -221.1815) ccw projected
  line L23 (-413.1791, -221.5813) -> (-181.0358, -47.3081) projected
  arc A68 (-181.0358, -47.3081) -> (-186.2425, -41.2134) centre (-183.8101, -44.4068) ccw projected
  line L24 (-186.2425, -41.2134) -> (-394.0669, -199.5107) projected
  arc A69 (-400.8847, -197.8054) -> (-394.0669, -199.5107) centre (-396.7936, -195.9309) ccw projected
  circle A70 centre (-209.3341, -63.7077) radius 1.5 projected
  circle A71 centre (-183.8101, -44.4068) radius 1.5 projected
  circle A72 centre (-243.8473, -90.7103) radius 1.5 projected
  circle A73 centre (-263.8405, -105.7194) radius 1.5 projected
  circle A74 centre (-299.8281, -132.7359) radius 1.5 projected
  circle A75 centre (-339.8144, -162.7542) radius 1.5 projected
  circle A76 centre (-379.8007, -192.7724) radius 1.5 projected
  circle A77 centre (-399.7939, -207.7816) radius 1.5 projected
  circle A78 centre (-359.8076, -177.7633) radius 1.5 projected
  circle A79 centre (-319.8213, -147.745) radius 1.5 projected
  circle A80 centre (-283.8336, -120.7286) radius 1.5 projected
  circle A81 centre (-223.8542, -75.7012) radius 1.5 projected
  point P0 (0, 0)
sketch "スケッチ17" plane through (0, 0, 6) normal (0, 0, 1) x (1, 0, 0)
  circle A0 centre (-299.8281, -132.7359) radius 1.5 projected
  point P0 (0, 0)
equation "\"d16\" = d15"
equation "\"d17\" = d16"
equation "\"d18\" = d17"
equation "\"d19\" = d18"
equation "\"d55\" = d54"
equation "\"d56\" = d55"
equation "\"d57\" = d56"
equation "\"d54\" = 25"
